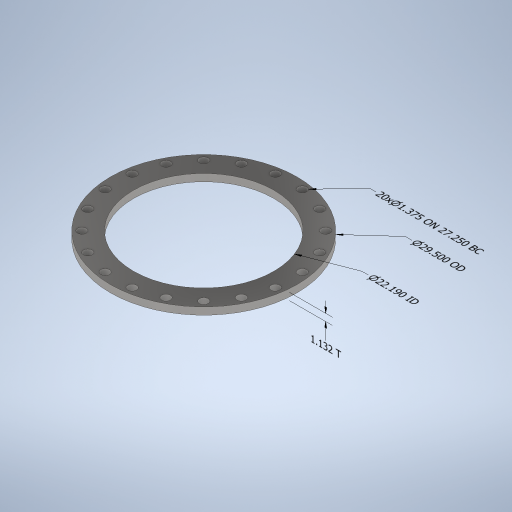
# Autodesk Inventor part: AWWA C207-18 Class B Ring and Blind Flange
Saved by Autodesk Inventor 2023 (Build 270158000, 158)
## iProperties
RuleStatus: InUse
Created: 2023-06-05
Part Number: AWWA C207-18 Class B Ring and Blind Flange
Material: Generic
Document SubType Name: Modeling
Designer: Admin
Density: 1 g/cm^3
Appearance: Steel - Polished
Author: Admin
Autodesk Inventor part; units mm, degrees
ref_plane "YZ Plane" through (0, 0, 0) normal (1, 0, 0) x (0, 1, 0)
ref_plane "XZ Plane" through (0, 0, 0) normal (0, 1, 0) x (-1, 0, 0)
ref_plane "XY Plane" through (0, 0, 0) normal (0, 0, 1) x (1, 0, 0)
sketch "Flange Sketch" plane through (0, 0, 0) normal (0, 1, 0) x (-1, 0, 0)
  circle A0 centre (0, 0) radius 374.65
  circle A1 centre (0, 0) radius 281.813
  circle A2 centre (0, 0) radius 346.075 construction
  line L0 (0, 0) -> (-54.1381, -341.8142) construction
  line L1 (0, 0) -> (0, -346.075) construction
  dimension "outerDiam" = 749.3
  dimension "innerDiam" = 563.626
  dimension "boltCircle" = 692.15
  dimension "boltOffsetAngle" = 9
  constraints: 4 end point, 3 centre point, 3 coincident, 2 point on circle, 1 vertical
  measures "outerDiam" diameter of A0
  measures "innerDiam" diameter of A1
  measures "boltCircle" diameter of A2
  measures "boltOffsetAngle" angle of L0 L1
extrude "Flange Extrusion" add sketch "Flange Sketch" along normal blind 28.7528
hole "Bolt Hole" at (54.1381, 0, -341.8142) direction (0, 1, 0) diameter 34.925 depth 28.7528
pattern_circular "Bolt Hole Pattern" count 20 over 360 about axis through (0, -10, 0) along (0, 1, 0) of "Bolt Hole"
equation "\"nominalSize\" = 558.8"
body "Solid1"
